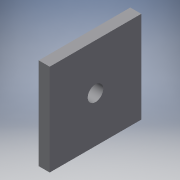
# Autodesk Inventor part: Top Plate
Saved by Autodesk Inventor 2019 (Build 230136000, 136)
## iProperties
Created: 2020-02-21
Part Number: Top Plate
Material: Generic
Document SubType Name: Modeling
Designer: ntb11189
Density: 1 g/cm^3
Appearance: Default
Author: ntb11189
Autodesk Inventor part; units mm, degrees
ref_plane "YZ Plane" through (0, 0, 0) normal (1, 0, 0) x (0, 1, 0)
ref_plane "XZ Plane" through (0, 0, 0) normal (0, 1, 0) x (-1, 0, 0)
ref_plane "XY Plane" through (0, 0, 0) normal (0, 0, 1) x (1, 0, 0)
sketch "Sketch1" plane through (0, 0, 0) normal (1, 0, 0) x (0, 1, 0)
  line L0 (0, 0) -> (-40, 0)
  line L1 (-40, 0) -> (-40, -40)
  line L2 (-40, -40) -> (0, -40)
  line L3 (0, -40) -> (0, 0)
  circle A0 centre (-20, -20) radius 3.4
  dimension "d0" = 40
  dimension "d1" = 40
  dimension "d2" = 3.4
  dimension "d3" = 20
  dimension "d4" = 20
  constraints: 8 end point, 2 parallel, 1 centre point, 1 horizontal, 1 perpendicular
  measures "d0" distance of L2.end L1.end
  measures "d1" distance of L1.end L0.end
  measures "d2" radius of A0
  measures "d3" distance from line of L3 A0.centre
  measures "d4" distance from line of L2 A0.centre
extrude "Extrusion1" add sketch "Sketch1" along normal blind 4.8
body "Solid1"
